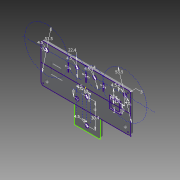
# Autodesk Inventor part: OuterBar
Saved by Autodesk Inventor 2014 SP1 (Build 180222100, 222)
## iProperties
Created: 2014-06-07
Part Number: OuterBar
Material: Generic
Document SubType Name: Modeling
Designer: Erin
Density: 1 g/cm^3
Appearance: Default
Author: Erin
Autodesk Inventor part; units mm, degrees
ref_plane "YZ Plane" through (0, 0, 0) normal (1, 0, 0) x (0, 1, 0)
ref_plane "XZ Plane" through (0, 0, 0) normal (0, 1, 0) x (-1, 0, 0)
ref_plane "XY Plane" through (0, 0, 0) normal (0, 0, 1) x (1, 0, 0)
sketch "Sketch1" plane through (0, 0, 0) normal (0, 1, 0) x (-1, 0, 0)
  line L0 (-51.65, 23.5) -> (51.65, 23.5)
  line L1 (54.65, 20.5) -> (54.65, -20.5)
  line L2 (51.65, -23.5) -> (-51.65, -23.5)
  line L3 (-54.65, -20.5) -> (-54.65, 20.5)
  circle A0 centre (-47.65, 16.5) radius 2.25
  circle A1 centre (47.65, 16.5) radius 2.25
  circle A2 centre (-47.65, 16.5) radius 26.75 construction
  circle A3 centre (-10.7, 16.5) radius 2.25
  circle A4 centre (-10.7, 16.5) radius 11.2 construction
  line L4 (-21.9, 16.5) -> (-21.9, 6.8604)
  line L5 (-20.9, 16.5) -> (-20.9, 6.8604)
  circle A5 centre (10.7, 16.5) radius 2.25
  circle A6 centre (10.7, 16.5) radius 11.2 construction
  line L6 (-0.5, 16.5) -> (-0.5, 5.694)
  line L7 (0.5, 16.5) -> (0.5, 5.694)
  circle A7 centre (47.65, 16.5) radius 26.75 construction
  line L8 (20.9, 16.5) -> (20.9, 5.8426)
  line L9 (21.9, 16.5) -> (21.9, 5.8426)
  arc A8 (-51.65, 23.5) -> (-54.65, 20.5) centre (-51.65, 20.5) ccw
  arc A9 (-54.65, -20.5) -> (-51.65, -23.5) centre (-51.65, -20.5) ccw
  arc A10 (54.65, 20.5) -> (51.65, 23.5) centre (51.65, 20.5) ccw
  arc A11 (51.65, -23.5) -> (54.65, -20.5) centre (51.65, -20.5) ccw
  line L10 (-84.9483, 16.5) -> (77.5332, 16.5) construction
  line L11 (-54.65, 0) -> (54.65, 0)
  line L12 (10.7, 30.5) -> (10.7, -33.5) construction
  circle A12 centre (10.7, -16.5) radius 2.25
  line L13 (5, -8.5) -> (18, -8.5) construction
  line L14 (3.7, -4.5) -> (3.7, -33.5) construction
  line L15 (-6.3, -4.5) -> (-6.3, -33.5) construction
  line L16 (-1.3, -33.5) -> (-1.3, -4.5) construction
  circle A13 centre (-1.3, -38.9) radius 2.25
  circle A14 centre (-1.3, -8.5) radius 2.25
  line L17 (-17.7373, -23.5) -> (14.2274, -23.5)
  line L18 (14.2274, -23.5) -> (14.2274, -45.3565)
  line L19 (14.2274, -45.3565) -> (-17.7373, -45.3565)
  line L20 (-17.7373, -45.3565) -> (-17.7373, -23.5)
  line L21 (-40.65, 5) -> (-30.65, 5)
  line L22 (-30.65, 5) -> (-30.65, -5)
  line L23 (-30.65, -5) -> (-40.65, -5)
  line L24 (-40.65, -5) -> (-40.65, 5)
  line L25 (-42.65, -7) -> (-28.65, -7)
  line L26 (-28.65, -7) -> (-28.65, 7)
  line L27 (-28.65, 7) -> (-42.65, 7)
  line L28 (-42.65, 7) -> (-42.65, -7)
  point P0 (0, 0)
  point P1 (-54.65, 23.5)
  point P2 (-54.65, -23.5)
  point P3 (0, 23.5)
  point P4 (-35.65, 5)
  point P5 (-30.65, 0)
  dimension "d5" = 53.5
  dimension "d12" = 53.5
  dimension "d1" = 4.5
  dimension "d2" = 7
  dimension "d3" = 4.5
  dimension "d4" = 7
  dimension "d6" = 4.5
  dimension "d7" = 22.4
  dimension "d8" = 1
  dimension "d9" = 4.5
  dimension "d10" = 22.4
  dimension "d11" = 1
  dimension "d13" = 1
  dimension "d14" = 3
  dimension "d23" = 16.5
  dimension "d24" = 7
  dimension "d27" = 8
  dimension "d28" = 7
  dimension "d29" = 10
  dimension "d30" = 5
  dimension "d31" = 4.5
  dimension "d32" = 4.5
  dimension "d33" = 30.4
  dimension "d38" = 0
  dimension "d40" = 10
  dimension "d41" = 10
  dimension "d43" = 2
  dimension "d47" = 12
  constraints: 58 end point, 17 parallel, 13 centre point, 12 point on circle, 12 point on line, 12 tangent, 8 perpendicular, 5 midpoint, 4 coincident, 4 horizontal alignment, 3 equal radius, 3 horizontal, 2 vertical, 1 symmetric about line, 1 vertical alignment, 8 other
  measures "d1" diameter of A0
  measures "d2" distance from line of A0.centre L3
  measures "d3" diameter of A1
  measures "d4" distance from line of A1.centre L1
  measures "d6" diameter of A3
  measures "d7" diameter of A4
  measures "d8" distance between parallel lines of L5 L4
  measures "d9" diameter of A5
  measures "d10" diameter of A6
  measures "d11" distance between parallel lines of L7 L6
  measures "d13" distance between parallel lines of L9 L8
  measures "d14" radius of A8
  measures "d23" distance between parallel lines of L11 L10
  measures "d24" distance between parallel lines of L10 L0
  measures "d27" distance from line of A12.centre L13
  measures "d28" distance between parallel lines of L14 L12
  measures "d29" distance between parallel lines of L15 L14
  measures "d30" distance between parallel lines of L14 L16
  measures "d31" diameter of A13
  measures "d32" diameter of A14
  measures "d33" distance of A13.centre A14.centre
  measures "d38" distance from line of A14.centre L13
  measures "d40" distance of L23.end L21.start
  measures "d41" distance of L21.start L21.end
  measures "d43" distance between parallel lines of L25 L23
  measures "d47" horizontal distance of point (-35.65, 5) A0.centre
extrude "Extrusion1" add sketch "Sketch1" along normal blind 3 contours L0 A10 L1 L11 L26 L27 L28 L3 A8 | L11 L28 L25 L26 L1 A11 L2 A9 L3 | L28 L27 L26 L11 L22 L21 L24 | L11 L24 L23 L22 L26 L25 L28 | L24 L21 L22 L11 | L11 L22 L23 L24 | A0 | A1 | A3 | A5 | A12 | A14
extrude "Extrusion2" cut sketch "Sketch1" along normal blind 10 contours A0 | A1 | A3 | A5
mirror "Mirror1" about plane through (0, 0, 0) normal (0, 0, 1) of "Extrusion2"
extrude "Extrusion3" add sketch "Sketch1" along normal blind 3 contours L2 L18 L19 L20
extrude "Extrusion4" cut sketch "Sketch1" along normal blind 3 contours A14
fillet "Fillet1" radius 3 2 edges at (-14.2274, 1.5, -45.3565) (17.7373, 1.5, -45.3565)
extrude "Extrusion5" cut sketch "Sketch1" along normal blind 1 contours L28 L27 L26 L11 L22 L21 L24 | L11 L24 L23 L22 L26 L25 L28
mirror "Mirror2" about plane through (0, 0, 0) normal (1, 0, 0) of "Extrusion5"
body "Solid1"
